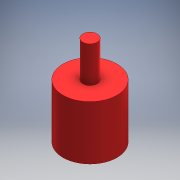
# Autodesk Inventor part: 防振ゴム雄ねじ雌ねじm4スペーサー長さ15
Saved by Autodesk Inventor 2020.2 (Build 242310000, 310)
## iProperties
Created: 2019-11-20
Part Number: 防振ゴム雄ねじ雌ねじm4スペーサー長さ15
Material: 一般
Document SubType Name: Modeling
Designer: mozar
Mass: 6 g
Surface Area: 12.2885 cm^2
Volume: 2.73934 cm^3
Density: 2.19031 g/cm^3
Appearance: 淡い赤
Author: mozar
Autodesk Inventor part; units mm, degrees
ref_plane "YZ Plane" through (0, 0, 0) normal (1, 0, 0) x (0, 1, 0)
ref_plane "XZ Plane" through (0, 0, 0) normal (0, 1, 0) x (-1, 0, 0)
ref_plane "XY Plane" through (0, 0, 0) normal (0, 0, 1) x (1, 0, 0)
sketch "スケッチ1" plane through (0, 0, 0) normal (0, 0, 1) x (1, 0, 0)
  circle A0 centre (0, 0) radius 7.5
  circle A1 centre (0, 0) radius 2
  dimension "d0" = 15
  dimension "d1" = 4
  constraints: 2 centre point, 2 coincident
  measures "d0" diameter of A0
  measures "d1" diameter of A1
extrude "押し出し1" add sketch "スケッチ1" along normal blind 10 contours A1
extrude "押し出し2" add sketch "スケッチ1" against normal blind 15 contours A0 | A1
sketch "スケッチ2" plane through (0, 0, -15) normal (0, 0, -1) x (-1, 0, 0)
  circle A0 centre (0, 0) radius 7.5 projected
hole "穴1" at (0, 0, -15) direction (0, 0, 1) diameter 3.3 depth 4 tip angle 118
